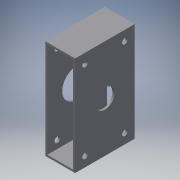
# Autodesk Inventor part: transmition Axle Support
Saved by Autodesk Inventor 2019 (Build 230136000, 136)
## iProperties
Created: 2019-10-21
Part Number: transmition Axle Support
Material: Generic
Document SubType Name: Modeling
Designer: admin
Density: 1 g/cm^3
Appearance: Default
Author: admin
Autodesk Inventor part; units mm, degrees
ref_plane "YZ Plane" through (0, 0, 0) normal (1, 0, 0) x (0, 1, 0)
ref_plane "XZ Plane" through (0, 0, 0) normal (0, 1, 0) x (-1, 0, 0)
ref_plane "XY Plane" through (0, 0, 0) normal (0, 0, 1) x (1, 0, 0)
sketch "Sketch1" plane through (0, 0, 0) normal (0, 0, 1) x (1, 0, 0)
  line L0 (-15, -50) -> (15, -50)
  line L1 (15, -50) -> (15, 50)
  line L2 (15, 50) -> (-15, 50)
  line L3 (-15, 50) -> (-15, -50)
  line L4 (-15, -50) -> (15, 50) construction
  line L5 (15, -50) -> (-15, 50) construction
  line L6 (-13, 48) -> (13, 48)
  line L7 (13, 48) -> (13, -48)
  line L8 (13, -48) -> (-13, -48)
  line L9 (-13, -48) -> (-13, 48)
  point P0 (0, 0)
  dimension "d0" = 30
  dimension "d1" = 100
  dimension "d2" = 2
  constraints: 20 end point, 4 parallel, 2 midpoint, 2 perpendicular, 1 horizontal, 3 other
  measures "d0" distance of L2.end L1.end
  measures "d1" distance of L1.end L0.end
  measures "d2" distance between parallel lines of L2 L6
extrude "Extrusion1" add sketch "Sketch1" along normal blind 60
sketch "Sketch2" plane through (15, -50, 0) normal (1, 0, 0) x (0, 0, -1)
  circle A0 centre (-30, 50) radius 9.65
  line L0 (-30, 100) -> (-30, 50) construction
  line L1 (0, 0) -> (0, 100) projected
  line L2 (0, 100) -> (-60, 100) projected
  line L3 (-30, 50) -> (0, 50) construction
  circle A1 centre (-50, 90) radius 2.75
  circle A2 centre (-10, 90) radius 2.75
  circle A3 centre (-20, 10) radius 2.75
  circle A4 centre (-50, 10) radius 2.75
  line L4 (0, 0) -> (-60, 0) projected
  dimension "d5" = 19.3
  dimension "d11" = 50
  dimension "d12" = 30
  dimension "d13" = 5.5
  dimension "d14" = 5.5
  dimension "d15" = 5.5
  dimension "d16" = 5.5
  dimension "d18" = 40
  dimension "d19" = 20
  dimension "d20" = 40
  dimension "d21" = 10
  dimension "d22" = 80
  dimension "d23" = 80
  dimension "d24" = 30
  dimension "d25" = 40
  constraints: 5 centre point, 4 end point, 1 horizontal, 1 midpoint, 1 vertical
  measures "d5" diameter of A0
  measures "d11" distance from line of L2 L0.end
  measures "d12" distance from line of L1 L0.end
  measures "d13" diameter of A1
  measures "d14" diameter of A2
  measures "d15" diameter of A3
  measures "d16" diameter of A4
  measures "d18" vertical distance of L0.end A4.centre
  measures "d19" horizontal distance of A4.centre L0.end
  measures "d20" vertical distance of A3.centre L0.end
  measures "d21" horizontal distance of A3.centre L0.end
  measures "d22" vertical distance of A2.centre A3.centre
  measures "d23" distance of A4.centre A1.centre
  measures "d24" horizontal distance of A3.centre A1.centre
  measures "d25" horizontal distance of A4.centre A2.centre
extrude "Extrusion2" cut sketch "Sketch2" against normal blind 38.5
sketch "Sketch3" plane through (-13, -48, 0) normal (1, 0, 0) x (0, 0, -1)
  circle A0 centre (-30, 48) radius 9.65 projected
  circle A1 centre (-30, 48) radius 15
  point P0 (0, 48)
  dimension "d8" = 30
  constraints: 1 centre point, 1 coincident
  measures "d8" diameter of A1
extrude "Extrusion3" cut sketch "Sketch3" against normal blind 2 contours A0 | A1
body "Solid1"
